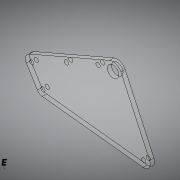
# Autodesk Inventor part: 中間外フレーム2
Saved by Autodesk Inventor 2019 (Build 230136000, 136)
## iProperties
Created: 2019-11-12
Part Number: 中間外フレーム2
Material: ポリカーボネート、クリア
Document SubType Name: Modeling
Designer: tanjihayato
Density: 1.2 g/cm^3
Appearance: ポリカーボネート - クリア
Mass: 10.1643 g
Surface Area: 64.8195 cm^2
Volume: 8.47028 cm^3
Author: tanjihayato
Autodesk Inventor part; units mm, degrees
ref_plane "YZ Plane" through (0, 0, 0) normal (1, 0, 0) x (0, 1, 0)
ref_plane "XZ Plane" through (0, 0, 0) normal (0, 1, 0) x (-1, 0, 0)
ref_plane "XY Plane" through (0, 0, 0) normal (0, 0, 1) x (1, 0, 0)
sketch "スケッチ1" plane through (0, 0, 0) normal (0, 0, 1) x (1, 0, 0)
  circle A0 centre (0, 0) radius 20.55 construction
  circle A1 centre (-21.6908, -16.4118) radius 19.1 construction
  circle A2 centre (25.3202, -9.9362) radius 19.1 construction
  circle A3 centre (-50.601, 30.8143) radius 1.5
  circle A4 centre (5.9362, 53.5882) radius 1.5
  circle A5 centre (27.3908, 10.6821) radius 1.5
  circle A6 centre (-42.8914, 18.3887) radius 1.5
  circle A7 centre (-21.6908, -16.4118) radius 4.025
  circle A8 centre (25.3202, -9.9362) radius 4.025
  circle A9 centre (0, 0) radius 4
  line L0 (-17.8785, -18.8026) -> (-30.4168, -38.7963) construction
  arc A10 (-17.8785, -18.8026) -> (-19.2493, -12.6317) centre (-21.6908, -16.4118) ccw construction
  line L1 (-19.2493, -12.6317) -> (-39.0737, 0.1727) construction
  line L2 (37.1409, -30.8522) -> (21.8866, -12.8448) construction
  arc A11 (22.3659, -6.5417) -> (21.8866, -12.8448) centre (25.3202, -9.9362) ccw construction
  line L3 (22.3659, -6.5417) -> (40.1678, 8.9519) construction
  line L4 (-21.6908, -16.4118) -> (-99.9742, 13.5882) construction
  line L5 (-105.5257, -16.4118) -> (-21.6908, -16.4118) construction
  line L6 (-21.6908, -16.4118) -> (-101.7113, -41.4118) construction
  line L7 (25.3202, -9.9362) -> (102.5386, -46.4118) construction
  line L8 (110.4743, -16.4118) -> (25.3202, -9.9362) construction
  line L9 (25.3202, -9.9362) -> (108.6869, 8.5882) construction
  line L10 (-18.0583, -13.7557) -> (-31.9879, 5.2949) construction
  line L11 (-17.339, -17.5569) -> (-24.5367, -44.9106) construction
  line L12 (21.5077, -7.5456) -> (34.045, 12.4488) construction
  line L13 (21.0739, -11.4259) -> (31.6059, -41.446) construction
  arc A12 (-24.6176, -40.3201) -> (-19.5065, -44.4166) centre (-20.132, -39.9603) ccw
  circle A13 centre (-20.132, -39.9603) radius 3 construction
  arc A14 (-38.9879, 7.9907) -> (-39.3359, 8.5262) centre (-35.3982, 10.7044) ccw construction
  circle A15 centre (-35.3982, 10.7044) radius 3 construction
  arc A16 (-31.9879, 5.2949) -> (-33.8465, 6.7744) centre (-35.6204, 2.6388) ccw construction
  circle A17 centre (-41.5152, -3.6073) radius 1.5
  line L14 (-33.8465, 6.7744) -> (-56.066, 16.3055) construction
  line L15 (-41.3386, 0.8892) -> (-72.6317, 2.1181) construction
  circle A18 centre (-42.8914, 18.3887) radius 3 construction
  circle A19 centre (-35.3982, 10.7044) radius 1.5
  circle A20 centre (36.7736, 17.5344) radius 1.5
  arc A21 (40.7942, 15.5132) -> (40.1934, 20.4593) centre (36.7736, 17.5344) ccw
  circle A22 centre (25.6508, -33.5339) radius 1.5
  arc A23 (26.2763, -37.9902) -> (30.1508, -33.5178) centre (25.6508, -33.5339) ccw
  circle A24 centre (36.7736, 17.5344) radius 3 construction
  circle A25 centre (25.6508, -33.5339) radius 3 construction
  arc A26 (36.6836, 14.4025) -> (34.045, 12.4488) centre (37.8575, 10.0583) ccw construction
  line L16 (36.6836, 14.4025) -> (64.1968, 21.8369) construction
  line L17 (43.2599, 10.0553) -> (82.9273, 8.8396) construction
  circle A27 centre (27.3908, 10.6821) radius 3 construction
  circle A28 centre (-21.6908, -16.4118) radius 7.025 construction
  circle A29 centre (25.3202, -9.9362) radius 7.025 construction
  arc A30 (40.8593, 15.6483) -> (30.1508, -33.5178) centre (146.4685, -33.1029) ccw
  arc A31 (-24.6176, -40.3201) -> (-39.1827, 8.2484) centre (-145.1158, -49.988) ccw
  arc A32 (-52.2824, 34.9884) -> (-54.1907, 28.1005) centre (-50.601, 30.8143) ccw
  arc A33 (9.356, 56.5132) -> (4.2549, 57.7623) centre (5.9362, 53.5882) ccw
  line L18 (-39.1827, 8.2484) -> (-54.1907, 28.1005)
  line L19 (-52.2824, 34.9884) -> (4.2549, 57.7623)
  line L20 (9.356, 56.5132) -> (40.1934, 20.4593)
  line L21 (-19.5065, -44.4166) -> (26.2763, -37.9902)
  circle A34 centre (-20.132, -39.9603) radius 1.5
  line L22 (-23.8868, -42.4405) -> (-17.339, -17.5569)
  arc A35 (-17.339, -17.5569) -> (-18.0583, -13.7557) centre (-21.6908, -16.4118) ccw
  line L23 (-18.0583, -13.7557) -> (-31.9879, 5.2949)
  arc A36 (-31.9879, 5.2949) -> (-33.8465, 6.7744) centre (-35.6204, 2.6388) ccw
  line L24 (-33.8465, 6.7744) -> (-40.0946, 9.4545)
  line L25 (40.7974, 15.5141) -> (36.6836, 14.4025)
  arc A37 (36.6836, 14.4025) -> (34.045, 12.4488) centre (37.8575, 10.0583) ccw
  line L26 (34.045, 12.4488) -> (21.5077, -7.5456)
  arc A38 (21.5077, -7.5456) -> (21.0739, -11.4259) centre (25.3202, -9.9362) ccw
  line L27 (21.0739, -11.4259) -> (29.592, -35.7057)
  dimension "d0" = 8.05
  dimension "d1" = 8.05
  dimension "d2" = 8
  dimension "d3" = 20.968
  dimension "d4" = 20.968
  dimension "d5" = 17.35
  dimension "d6" = 17.35
  dimension "d7" = 16.877
  dimension "d8" = 16.877
  dimension "d9" = 20.936
  dimension "d10" = 20.936
  dimension "d11" = 9
  dimension "d12" = 6
  dimension "d13" = 9
  dimension "d14" = 6
  dimension "d15" = 9
  dimension "d16" = 20.968
  dimension "d17" = 20.968
  dimension "d18" = 6
  dimension "d19" = 3
  dimension "d20" = 3
  dimension "d21" = 9
  dimension "d22" = 3
  dimension "d23" = 9
  dimension "d24" = 6
  dimension "d25" = 6
  dimension "d26" = 9
  dimension "d27" = 16.877
  dimension "d28" = 3
  dimension "d29" = 3
  dimension "d30" = 9
  dimension "d31" = 9
  dimension "d32" = 3
  constraints: 56 end point, 40 point on circle, 39 centre point, 31 tangent, 14 coincident, 6 point on line, 2 equal length, 1 collinear, 1 concentric
  measures "d0" diameter of A7
  measures "d1" diameter of A8
  measures "d2" diameter of A9
  measures "d3" angle of L5 L4
  measures "d4" angle of L1 L10
  measures "d5" angle of L5 L6
  measures "d6" angle of L0 L11
  measures "d7" angle of L8 L9
  measures "d8" angle of L12 L3
  measures "d9" angle of L8 L7
  measures "d10" angle of L13 L2
  measures "d11" diameter of A12
  measures "d12" diameter of A13
  measures "d13" diameter of A14
  measures "d14" diameter of A15
  measures "d15" diameter of A16
  measures "d17" angle of L15 L14
  measures "d18" diameter of A18
  measures "d19" diameter of A19
  measures "d20" diameter of A20
  measures "d21" diameter of A21
  measures "d22" diameter of A22
  measures "d23" diameter of A23
  measures "d24" diameter of A24
  measures "d25" diameter of A25
  measures "d26" diameter of A26
  measures "d27" angle of L16 L17
  measures "d28" radial gap between concentric circles of A7 A28
  measures "d29" radial gap between concentric circles of A8 A29
  measures "d30" diameter of A32
  measures "d31" diameter of A33
  measures "d32" diameter of A34
sketch "スケッチ2" plane through (0, 0, 0) normal (0, 0, 1) x (1, 0, 0)
  circle A0 centre (-50.601, 30.8143) radius 1.5 projected
  circle A1 centre (-42.8914, 18.3887) radius 1.5 projected
  circle A2 centre (5.9362, 53.5882) radius 1.5 projected
  circle A3 centre (27.3908, 10.6821) radius 1.5 projected
  arc A4 (-52.3846, 34.9457) -> (-54.4248, 28.4418) centre (-50.601, 30.8143) ccw
  arc A5 (-46.7151, 16.0162) -> (-43.3819, 13.9155) centre (-42.8914, 18.3887) ccw
  arc A6 (11.384, 56.1025) -> (3.5581, 59.0968) centre (5.9362, 53.5882) ccw
  arc A7 (26.9003, 6.2089) -> (31.4766, 12.5678) centre (27.3908, 10.6821) ccw
  line L0 (-46.7151, 16.0162) -> (-54.4248, 28.4418)
  line L1 (-52.3846, 34.9457) -> (3.5581, 59.0968)
  line L2 (11.384, 56.1025) -> (31.4766, 12.5678)
  line L3 (26.9003, 6.2089) -> (-43.3819, 13.9155)
  circle A8 centre (5.9362, 53.5882) radius 4.025
  point P0 (0, 0)
  dimension "d33" = 3
  dimension "d34" = 3
  dimension "d35" = 4.5
  dimension "d36" = 3
  dimension "d39" = 8.05
  constraints: 8 end point, 8 point on circle, 8 tangent, 5 centre point, 1 coincident
  measures "d33" radial gap between concentric circles of A0 A4
  measures "d34" radial gap between concentric circles of A1 A5
  measures "d35" radial gap between concentric circles of A2 A6
  measures "d36" radial gap between concentric circles of A3 A7
  measures "d39" diameter of A8
extrude "押し出し1" add sketch "スケッチ2" along normal blind 3 contours L1 A6 L2 A7 L3 A5 L0 A4
sketch "スケッチ3" plane through (0, 0, 3) normal (0, 0, 1) x (1, 0, 0)
  circle A0 centre (5.9362, 53.5882) radius 4.025 projected
  circle A1 centre (27.3908, 10.6821) radius 1.5 projected
  circle A2 centre (-42.8914, 18.3887) radius 1.5 projected
  circle A3 centre (-50.601, 30.8143) radius 1.5 projected
  line L0 (-54.4248, 28.4418) -> (-46.7151, 16.0162) projected
  arc A4 (-46.7151, 16.0162) -> (-43.3819, 13.9155) centre (-42.8914, 18.3887) ccw projected
  line L1 (-43.3819, 13.9155) -> (26.9003, 6.2089) projected
  arc A5 (26.9003, 6.2089) -> (31.4766, 12.5678) centre (27.3908, 10.6821) ccw projected
  line L2 (31.4766, 12.5678) -> (11.384, 56.1025) projected
  arc A6 (11.384, 56.1025) -> (3.5581, 59.0968) centre (5.9362, 53.5882) ccw projected
  line L3 (3.5581, 59.0968) -> (-52.3846, 34.9457) projected
  arc A7 (-52.3846, 34.9457) -> (-54.4248, 28.4418) centre (-50.601, 30.8143) ccw projected
  circle A8 centre (5.9362, 53.5882) radius 6
  circle A9 centre (-26.5254, 42.8418) radius 1.5
  circle A10 centre (-4.491, 52.3543) radius 1.5
  circle A11 centre (-4.491, 52.3543) radius 4.5 construction
  point P0 (0, 0)
  dimension "d40" = 12
  dimension "d41" = 3
  dimension "d42" = 3
  dimension "d43" = 3
  dimension "d44" = 3
  dimension "d45" = 24
  dimension "d46" = 9
  constraints: 4 centre point, 2 coincident, 1 tangent
  measures "d40" diameter of A8
  measures "d41" diameter of A9
  measures "d42" diameter of A10
  measures "d43" distance from line of L3 A10.centre
  measures "d44" distance from line of L3 A9.centre
  measures "d45" distance of A9.centre A10.centre
  measures "d46" diameter of A11
extrude "押し出し2" cut sketch "スケッチ3" against normal blind 10 contours A9 | A10
equation "\"d4\" = d3"
equation "\"d6\" = d5"
equation "\"d8\" = d7"
equation "\"d10\" = d9"
equation "\"d16\" = d3"
equation "\"d17\" = d3"
equation "\"d27\" = d7"
